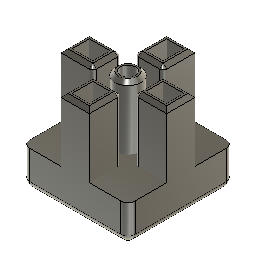
EXTRUSIONcap (Autodesk Fusion 360 design; units mm, degrees)
Autodesk Fusion 360 part; units mm, degrees
sketch "Sketch1" plane through (0, 0, 0) normal (0, 0, 1) x (1, 0, 0)
  line L0 (15, 15) -> (-15, 15)
  line L1 (-15, 15) -> (-15, -15)
  line L2 (-15, -15) -> (15, -15)
  line L3 (15, -15) -> (15, 15)
  line L4 (15, 15) -> (-15, -15) construction
  line L5 (-15, 15) -> (15, -15) construction
  line L6 (0, -15) -> (0, 15) construction
  line L7 (15, 0) -> (-15, 0) construction
  line L8 (-4, -15) -> (4, -15)
  line L9 (4, -15) -> (4, -6)
  line L10 (4, -6) -> (-4, -6)
  line L11 (-4, -6) -> (-4, -15)
  line L12 (-4, -15) -> (4, -6) construction
  line L13 (4, -15) -> (-4, -6) construction
  line L14 (6, -4) -> (15, -4)
  line L15 (6, 4) -> (6, -4)
  line L16 (15, 4) -> (6, 4)
  line L17 (4, 6) -> (4, 15)
  line L18 (-4, 6) -> (4, 6)
  line L19 (-4, 15) -> (-4, 6)
  line L20 (-6, 4) -> (-15, 4)
  line L21 (-6, -4) -> (-6, 4)
  line L22 (-15, -4) -> (-6, -4)
  circle A0 centre (0, 0) radius 3.65
  point P0 (0, -10.5)
  dimension "d13" = 30
  dimension "d14" = 30
  dimension "d19" = 8
  dimension "d20" = 9
  dimension "d22" = 360
  dimension "d23" = 7.3
  constraint horizontal L0
  constraint perpendicular L0 L1
  constraint parallel L0 L2
  constraint parallel L1 L3
  constraint coincident L4 A0.centre
  constraint coincident L5 A0.centre
  constraint coincident A0.centre origin
  constraint midpoint L2 L6.start
  constraint midpoint L0 L6.end
  constraint midpoint L3 L7.start
  constraint midpoint L1 L7.end
  constraint horizontal L8
  constraint perpendicular L8 L9
  constraint parallel L8 L10
  constraint parallel L9 L11
  constraint coincident L12 P0
  constraint coincident L13 P0
  constraint coincident L6 P0
  constraint collinear L2 L8
  measures "d13" distance of L1.end L2.end
  measures "d14" distance of L0.end L1.end
  measures "d19" distance of L9.end L10.end
  measures "d20" distance of L8.end L9.end
  measures "d23" diameter of A0
extrude "Extrude1" add sketch "Sketch1" along normal blind 10 contours L0 L1 L2 L3 L9 L10 L11 L14 L15 L16 L17 L18 L19 L20 L21 L22 | L0 L17 L18 L19 | L3 L14 L15 L16 | L1 L20 L21 L22 | L2 L8 L9 L10 L11 | A0 in component "foot"
extrude "Extrude2" add sketch "Sketch1" along normal blind 28 thin wall 1.5 inside contours L0 L17 L18 L19 | L3 L14 L15 L16 | L1 L20 L21 L22 | L2 L8 L9 L10 L11 | A0 in component "foot"
fillet "Fillet1" radius 2 4 edges at (-15, -15, 5) (15, -15, 5) (15, 15, 5) (-15, 15, 5) in component "foot"
fillet "Fillet1" radius 1 8 edges at (-6, -4, 19) (-6, 4, 19) (-4, 6, 19) (4, 6, 19) (6, -4, 19) (4, -6, 19) (-4, -6, 19) (6, 4, 19) in component "foot"
chamfer "Chamfer1" distance 1 angle 45 8 edges at (0, 15, 0) (-14.4142, 14.4142, 0) (-15, 0, 0) (-14.4142, -14.4142, 0) (0, -15, 0) (14.4142, -14.4142, 0) (15, 0, 0) (14.4142, 14.4142, 0) in component "foot"
chamfer "Chamfer1" distance 1 angle 45 25 edges at (11, -4, 28) (11, 4, 28) (6.2929, 3.7071, 28) (6, 0, 28) (6.2929, -3.7071, 28) (15, 0, 28) (4, -11, 28) (3.7071, -6.2929, 28) (0, -6, 28) (-3.7071, -6.2929, 28) (-4, -11, 28) (0, -15, 28) (-11, -4, 28) (-6.2929, -3.7071, 28) (-6, 0, 28) (-6.2929, 3.7071, 28) (-11, 4, 28) (-15, 0, 28) (-4, 11, 28) (-3.7071, 6.2929, 28) (0, 6, 28) (3.7071, 6.2929, 28) (4, 11, 28) (0, 15, 28) (-3.403, -1.3199, 28) in component "foot"
fillet "Fillet2" radius 2 8 edges at (14.4142, 14.4142, 1) (15, 0, 1) (14.4142, -14.4142, 1) (0, -15, 1) (-14.4142, -14.4142, 1) (-15, 0, 1) (-14.4142, 14.4142, 1) (0, 15, 1) in component "foot"
component "foot" placed x (1, 0, 0) y (0, 1, 0) z (0, 0, 1) at (0, 0, 0)
equation "d15 = height"
equation "d24 = height + 18 mm"
equation "height = 10 mm"
